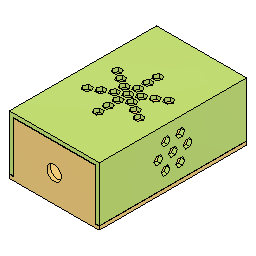
power-supply-case (Autodesk Fusion 360 design; units mm, degrees)
Autodesk Fusion 360 part; units mm, degrees
note: some values were not read from the file. Chosen so that the rebuilt part matches the saved one: which face or edge a step refers to. Set by a fixed rule: which sketch regions a step uses.
sketch "Sketch1" plane through (0, 0, 0) normal (0, 1, 0) x (1, 0, 0) in component "Bottom"
  line L0 (0, 0) -> (71, 0)
  line L1 (71, 0) -> (71, 116.4)
  line L2 (71, 116.4) -> (0, 116.4)
  line L3 (0, 116.4) -> (0, 0)
  dimension "d6" = 71
  dimension "d7" = 116.4
  dimension "d84" = 0
  dimension "d85" = 0
  dimension "d86" = 0
  dimension "d87" = 0
  constraint horizontal L0
  constraint vertical L1
  constraint horizontal L2
  constraint vertical L3
  constraint coincident L0.start L3.end
  measures "d6" distance of L0.start L0.end
  measures "d7" distance of L0.start L2.end
extrude "Extrude1" add sketch "Sketch1" along normal blind 42.8 makes body 1 in component "Bottom"
shell "Shell1" thickness 2.8 removed faces 1 at (23.6667, 42.8, -38.8) on bodies 1 in component "Bottom"
sketch "Sketch2" plane through (0, 42.8, 0) normal (0, 1, 0) x (-1, 0, 0) in component "Bottom"
  line L0 (-2.8, -113.6) -> (-68.2, -113.6)
  line L1 (-68.2, -113.6) -> (-68.2, -2.8)
  line L2 (-68.2, -2.8) -> (-2.8, -2.8)
  line L3 (-2.8, -2.8) -> (-2.8, -113.6)
  line L4 (0, -116.4) -> (0, 0)
  line L5 (0, 0) -> (-71, 0)
  line L6 (-71, 0) -> (-71, -116.4)
  line L7 (-71, -116.4) -> (0, -116.4)
  line L8 (0, -58.2) -> (-35.5, -58.2) construction
  line L9 (-67.9, 0) -> (-3.1, 0)
  line L10 (-3.1, 0) -> (-3.1, -116.4)
  line L11 (-3.1, -116.4) -> (-67.9, -116.4)
  line L12 (-67.9, -116.4) -> (-67.9, 0)
  line L13 (-67.9, 0) -> (-3.1, -116.4) construction
  line L14 (-3.1, 0) -> (-67.9, -116.4) construction
  point P0 (-35.5, -58.2)
  dimension "d11" = 35.5
  dimension "d12" = 116.4
  dimension "d13" = 64.8
  constraint horizontal L8
  constraint midpoint L4 L8.start
  constraint perpendicular L9 L10
  constraint parallel L9 L11
  constraint parallel L10 L12
  constraint horizontal L9
  constraint coincident L13 P0
  constraint coincident L14 P0
  constraint coincident P0 L8.end
  measures "d11" distance of L8.start P0
  measures "d12" distance of L9.end L10.end
  measures "d13" distance of L10.end L11.end
extrude "Extrude2" cut sketch "Sketch2" against normal blind 40 contours L0 L2 L3 L4 L5 L7 L10 | L0 L1 L2 L5 L6 L7 L12 bodies 1 in component "Bottom"
sketch "Sketch1 (2)" plane through (0, 42.8, 0) normal (0, 1, 0) x (-1, 0, 0) in component "Cover"
  line L0 (-3.1, -2.8) -> (-3.1, 0)
  line L1 (-3.1, 0) -> (-67.9, 0)
  line L2 (-67.9, 0) -> (-67.9, -2.8)
  line L3 (-67.9, -2.8) -> (-3.1, -2.8)
  line L4 (0, 0) -> (-71, 0)
  line L5 (-71, 0) -> (-71, -116)
  line L6 (-71, -116) -> (0, -116)
  line L7 (0, -116) -> (0, 0)
  dimension "d16" = 116
  dimension "d17" = 71
  dimension "d80" = 0
  dimension "d81" = 0
  dimension "d82" = 0
  dimension "d83" = 0
  constraint horizontal L4
  constraint vertical L5
  constraint horizontal L6
  constraint vertical L7
  constraint coincident L4.start L7.end
  measures "d16" distance of L4.start L6.end
  measures "d17" distance of L4.start L4.end
extrude "Extrude1'" add sketch "Sketch1 (2)" along normal blind 3 separate body makes body 2 in component "Cover"
sketch "Sketch2 (2)" plane through (0, 42.8, 0) normal (0, -1, 0) x (1, 0, 0) in component "Cover"
  line L0 (0, 0) -> (0, -116)
  line L1 (0, -116) -> (71, -116)
  line L2 (71, -116) -> (71, 0)
  line L3 (71, 0) -> (0, 0)
  line L4 (0, 0) -> (3, 0)
  line L5 (3, 0) -> (3, -116)
  line L6 (3, -116) -> (0, -116)
  line L7 (0, -116) -> (0, 0)
  line L8 (71, 0) -> (68, 0)
  line L9 (68, 0) -> (68, -116)
  line L10 (68, -116) -> (71, -116)
  line L11 (71, -116) -> (71, 0)
  dimension "d20" = 116
  dimension "d21" = 3
  dimension "d22" = 3
  dimension "d23" = 116
  constraint horizontal L4
  constraint vertical L5
  constraint horizontal L6
  constraint vertical L7
  constraint coincident L0.start L3.end
  constraint horizontal L8
  constraint vertical L9
  constraint horizontal L10
  constraint vertical L11
  constraint coincident L2.end L3.start
  measures "d20" distance of L0.start L0.end
  measures "d21" distance of L0.start L4.end
  measures "d22" distance of L2.end L8.end
  measures "d23" distance of L2.end L1.end
extrude "Extrude2'" add sketch "Sketch2 (2)" along normal blind 40 contours L0 L1 L3 L4 L5 L6 L7 | L1 L2 L3 L8 L9 L10 L11 bodies 2 in component "Cover"
sketch "Sketch2 (3)" plane through (68, 0, 0) normal (-1, 0, 0) x (0, 0, 1) in component "Cover"
  line L0 (0, 42.8) -> (-116, 42.8)
  line L1 (-116, 42.8) -> (-116, 2.8)
  line L2 (-116, 2.8) -> (0, 2.8)
  line L3 (0, 2.8) -> (0, 42.8)
  line L4 (-116, 42.8) -> (-113, 42.8) construction
  line L5 (-113, 42.8) -> (-110, 42.8)
  line L6 (-110, 42.8) -> (-110, 2.8)
  line L7 (-110, 2.8) -> (-113, 2.8)
  line L8 (-113, 2.8) -> (-113, 42.8)
  dimension "d26" = 3
  dimension "d27" = 3
  dimension "d28" = 40
  constraint coincident L0.end L1.start
  constraint perpendicular L1 L4
  constraint horizontal L5
  constraint vertical L6
  constraint horizontal L7
  constraint vertical L8
  measures "d26" distance of L0.end L4.end
  measures "d27" distance of L4.end L5.end
  measures "d28" distance of L4.end L7.end
extrude "Extrude3" add sketch "Sketch2 (3)" along normal blind 6 contours L0 L2 L5 L6 L7 L8 bodies 2 in component "Cover"
ref_plane "WorkPlane1" through (35.5, 24.3, -58) normal (0, 0, -1) x (-1, 0, 0) in component "Cover"
ref_plane "WorkPlane1" through (35.5, 22.8, -58) normal (-1, 0, 0) x (0, 0, -1) in component "Cover"
mirror "Mirror1" about plane through (35.5, 24.3, -58) normal (0, 0, -1) of "Extrude3" in component "Cover"
mirror "Mirror2" about plane through (35.5, 22.8, -58) normal (-1, 0, 0) of 6 faces at (62, 29.4667, -112) (66, 16.1333, -113) (66, 29.4667, -110) (66, 16.1333, -3) (62, 29.4667, -4) (66, 29.4667, -6) on bodies 2 in component "Cover"
chamfer "Chamfer1" distance 3 angle 45 2 edges at (68, 42.8, -58) (3, 42.8, -58) on bodies 2 in component "Cover"
chamfer "Chamfer2" distance 6 angle 45 4 edges at (68, 21.3, -6) (68, 21.3, -110) (3, 21.3, -110) (3, 21.3, -6) on bodies 2 in component "Cover"
chamfer "Chamfer1'" distance 3 angle 45 1 edges at (35.5, 2.8, -113.6) on bodies 1 in component "Bottom"
sketch "Sketch2 (1)" plane through (3.1, 0, 0) normal (-1, 0, 0) x (0, 0, 1) in component "Bottom"
  line L0 (-113.6, 5.8) -> (-113.6, 42.8)
  line L1 (-113.6, 42.8) -> (-116.4, 42.8)
  line L2 (-116.4, 2.8) -> (-110.6, 2.8)
  line L3 (-110.6, 2.8) -> (-113.6, 5.8)
  line L4 (-113.6, 5.8) -> (-113.6, 2.8)
  line L5 (-116.4, 42.8) -> (-116.4, 2.8)
  dimension "d36" = 3
  constraint vertical L4
  constraint coincident L0.start L3.end
  measures "d36" distance of L0.start L4.end
extrude "Extrude3'" cut sketch "Sketch2 (1)" against normal blind 7.5 contours L2 L3 L4 bodies 1 in component "Bottom"
sketch "Sketch3" plane through (67.9, 0, 0) normal (1, 0, 0) x (0, 0, -1) in component "Bottom"
  line L0 (110.6, 2.8) -> (116.4, 2.8)
  line L1 (116.4, 42.8) -> (113.6, 42.8)
  line L2 (113.6, 42.8) -> (113.6, 5.8)
  line L3 (113.6, 5.8) -> (110.6, 2.8)
  line L4 (113.6, 5.8) -> (113.6, 2.8)
  line L5 (116.4, 2.8) -> (116.4, 42.8)
  dimension "d39" = 3
  constraint vertical L4
  constraint coincident L2.end L3.start
  measures "d39" distance of L2.end L4.end
extrude "Extrude4" cut sketch "Sketch3" against normal blind 7.5 contours L0 L3 L4 bodies 1 in component "Bottom"
ref_plane "WorkPlane1" through (35.5, 22.8, -58.2) normal (0, 0, 1) x (1, 0, 0) in component "Bottom"
mirror "Mirror1'" about plane through (35.5, 22.8, -58.2) normal (0, 0, 1) of 3 faces at (43.8, 3.8, -111.6) (10.6, 3.8, -112.6) (60.4, 3.8, -112.6) on bodies 1 in component "Bottom"
sketch "Sketch4" plane through (0, 0, -116.4) normal (0, 0, -1) x (-1, 0, 0) in component "Bottom"
  line L0 (0, 2.8) -> (-3.1, 2.8)
  line L1 (-3.1, 2.8) -> (-3.1, 42.8)
  line L2 (-3.1, 42.8) -> (-67.9, 42.8)
  line L3 (-67.9, 42.8) -> (-67.9, 2.8)
  line L4 (-67.9, 2.8) -> (-71, 2.8)
  line L5 (-71, 2.8) -> (-71, 0)
  line L6 (-71, 0) -> (0, 0)
  line L7 (0, 0) -> (0, 2.8)
  line L8 (-18, 15.3) -> (-53, 15.3) construction
  line L9 (-53, 15.3) -> (-53, 30.3) construction
  line L10 (-53, 30.3) -> (-18, 30.3) construction
  line L11 (-18, 30.3) -> (-18, 15.3) construction
  line L12 (-18, 15.3) -> (-53, 30.3) construction
  line L13 (-53, 15.3) -> (-18, 30.3) construction
  line L14 (-30.4, 16.8) -> (-40.6, 16.8)
  line L15 (-45.6, 21.8) -> (-45.6, 23.8)
  line L16 (-40.6, 28.8) -> (-30.4, 28.8)
  line L17 (-25.4, 23.8) -> (-25.4, 21.8)
  line L18 (-25.4, 16.8) -> (-45.6, 28.8) construction
  line L19 (-45.6, 16.8) -> (-25.4, 28.8) construction
  arc A0 (-40.6, 28.8) -> (-45.6, 23.8) centre (-40.6, 23.8) ccw
  arc A1 (-25.4, 23.8) -> (-30.4, 28.8) centre (-30.4, 23.8) ccw
  arc A2 (-30.4, 16.8) -> (-25.4, 21.8) centre (-30.4, 21.8) ccw
  arc A3 (-45.6, 21.8) -> (-40.6, 16.8) centre (-40.6, 21.8) ccw
  line L20 (-67.9, 22.8) -> (-3.1, 22.8) construction
  point P0 (-35.5, 22.8)
  point P1 (-35.5, 22.8)
  dimension "d100" = 35
  dimension "d101" = 15
  dimension "d103" = 20.2
  dimension "d104" = 12
  dimension "d105" = 5
  constraint perpendicular L8 L9
  constraint parallel L8 L10
  constraint parallel L9 L11
  constraint horizontal L8
  constraint coincident L12 P1
  constraint coincident L13 P1
  constraint perpendicular L14 L15
  constraint parallel L14 L16
  constraint parallel L15 L17
  constraint horizontal L14
  constraint coincident L18 P1
  constraint coincident L19 P1
  constraint coincident P1 P0
  constraint coincident L18.end L15
  constraint coincident L18.end L16
  constraint tangent L15 A0
  constraint tangent L16 A0
  constraint coincident L19.end L16
  constraint coincident L19.end L17
  constraint tangent L16 A1
  constraint tangent L17 A1
  constraint equal A0 A1
  constraint coincident L18.start L14
  constraint coincident L18.start L17
  constraint tangent L14 A2
  constraint tangent L17 A2
  constraint equal A0 A2
  constraint coincident L19.start L14
  constraint coincident L19.start L15
  constraint tangent L14 A3
  constraint tangent L15 A3
  constraint equal A0 A3
  constraint midpoint L3 L20.start
  constraint midpoint L1 L20.end
  constraint midpoint P1 L20
  measures "d100" distance of L9.end L10.end
  measures "d101" distance of L8.end L9.end
  measures "d103" distance of L18.end L19.end
  measures "d104" distance of L19.start L18.end
  measures "d105" radius of A0
extrude "Extrude5" cut sketch "Sketch4" against normal up to surface (2.8 mm away) contours L14 L15 L16 L17 A0 A1 A2 A3 bodies 1 in component "Bottom"
sketch "Sketch3 (2)" plane through (0, 45.8, 0) normal (0, 1, 0) x (-1, 0, 0) in component "Cover"
  line L0 (0, -116) -> (0, 0)
  line L1 (0, 0) -> (-71, 0)
  line L2 (-71, 0) -> (-71, -116)
  line L3 (-71, -116) -> (0, -116)
  line L4 (-71, -58) -> (0, -58) construction
  line L5 (-35.5, -116) -> (-35.5, 0) construction
  line L6 (-38.9641, -58) -> (-37.2321, -61)
  line L7 (-37.2321, -61) -> (-33.7679, -61)
  line L8 (-33.7679, -61) -> (-32.0359, -58)
  line L9 (-32.0359, -58) -> (-33.7679, -55)
  line L10 (-33.7679, -55) -> (-37.2321, -55)
  line L11 (-37.2321, -55) -> (-38.9641, -58)
  line L12 (-38.0981, -59.5) -> (-40.6727, -60.9864) construction
  line L13 (-13.4164, -49.25) -> (-11.6843, -46.25)
  line L14 (-16.8805, -49.25) -> (-13.4164, -49.25)
  line L15 (-18.6125, -46.25) -> (-16.8805, -49.25)
  line L16 (-16.8805, -43.25) -> (-18.6125, -46.25)
  line L17 (-13.4164, -43.25) -> (-16.8805, -43.25)
  line L18 (-11.6843, -46.25) -> (-13.4164, -43.25)
  line L19 (-20.2002, -53.1667) -> (-18.4682, -50.1667)
  line L20 (-23.6643, -53.1667) -> (-20.2002, -53.1667)
  line L21 (-25.3964, -50.1667) -> (-23.6643, -53.1667)
  line L22 (-23.6643, -47.1667) -> (-25.3964, -50.1667)
  line L23 (-20.2002, -47.1667) -> (-23.6643, -47.1667)
  line L24 (-18.4682, -50.1667) -> (-20.2002, -47.1667)
  line L25 (-26.9841, -57.0833) -> (-25.252, -54.0833)
  line L26 (-30.4482, -57.0833) -> (-26.9841, -57.0833)
  line L27 (-32.1802, -54.0833) -> (-30.4482, -57.0833)
  line L28 (-30.4482, -51.0833) -> (-32.1802, -54.0833)
  line L29 (-26.9841, -51.0833) -> (-30.4482, -51.0833)
  line L30 (-25.252, -54.0833) -> (-26.9841, -51.0833)
  line L31 (-40.5518, -64.9167) -> (-38.8198, -61.9167)
  line L32 (-44.0159, -64.9167) -> (-40.5518, -64.9167)
  line L33 (-45.748, -61.9167) -> (-44.0159, -64.9167)
  line L34 (-44.0159, -58.9167) -> (-45.748, -61.9167)
  line L35 (-40.5518, -58.9167) -> (-44.0159, -58.9167)
  line L36 (-38.8198, -61.9167) -> (-40.5518, -58.9167)
  line L37 (-47.3357, -68.8333) -> (-45.6036, -65.8333)
  line L38 (-50.7998, -68.8333) -> (-47.3357, -68.8333)
  line L39 (-52.5318, -65.8333) -> (-50.7998, -68.8333)
  line L40 (-50.7998, -62.8333) -> (-52.5318, -65.8333)
  line L41 (-47.3357, -62.8333) -> (-50.7998, -62.8333)
  line L42 (-45.6036, -65.8333) -> (-47.3357, -62.8333)
  line L43 (-54.1195, -72.75) -> (-52.3875, -69.75)
  line L44 (-57.5836, -72.75) -> (-54.1195, -72.75)
  line L45 (-59.3157, -69.75) -> (-57.5836, -72.75)
  line L46 (-57.5836, -66.75) -> (-59.3157, -69.75)
  line L47 (-54.1195, -66.75) -> (-57.5836, -66.75)
  line L48 (-52.3875, -69.75) -> (-54.1195, -66.75)
  line L49 (-38.9641, -50.1667) -> (-37.2321, -53.1667)
  line L50 (-37.2321, -53.1667) -> (-33.7679, -53.1667)
  line L51 (-33.7679, -53.1667) -> (-32.0359, -50.1667)
  line L52 (-32.0359, -50.1667) -> (-33.7679, -47.1667)
  line L53 (-33.7679, -47.1667) -> (-37.2321, -47.1667)
  line L54 (-37.2321, -47.1667) -> (-38.9641, -50.1667)
  line L55 (-44.0159, -57.0833) -> (-40.5518, -57.0833)
  line L56 (-40.5518, -57.0833) -> (-38.8198, -54.0833)
  line L57 (-38.8198, -54.0833) -> (-40.5518, -51.0833)
  line L58 (-40.5518, -51.0833) -> (-44.0159, -51.0833)
  line L59 (-44.0159, -51.0833) -> (-45.748, -54.0833)
  line L60 (-45.748, -54.0833) -> (-44.0159, -57.0833)
  line L61 (-40.5518, -64.9167) -> (-38.8198, -61.9167)
  line L62 (-38.8198, -61.9167) -> (-40.5518, -58.9167)
  line L63 (-40.5518, -58.9167) -> (-44.0159, -58.9167)
  line L64 (-44.0159, -58.9167) -> (-45.748, -61.9167)
  line L65 (-45.748, -61.9167) -> (-44.0159, -64.9167)
  line L66 (-44.0159, -64.9167) -> (-40.5518, -64.9167)
  line L67 (-32.0359, -65.8333) -> (-33.7679, -62.8333)
  line L68 (-33.7679, -62.8333) -> (-37.2321, -62.8333)
  line L69 (-37.2321, -62.8333) -> (-38.9641, -65.8333)
  line L70 (-38.9641, -65.8333) -> (-37.2321, -68.8333)
  line L71 (-37.2321, -68.8333) -> (-33.7679, -68.8333)
  line L72 (-33.7679, -68.8333) -> (-32.0359, -65.8333)
  line L73 (-26.9841, -58.9167) -> (-30.4482, -58.9167)
  line L74 (-30.4482, -58.9167) -> (-32.1802, -61.9167)
  line L75 (-32.1802, -61.9167) -> (-30.4482, -64.9167)
  line L76 (-30.4482, -64.9167) -> (-26.9841, -64.9167)
  line L77 (-26.9841, -64.9167) -> (-25.252, -61.9167)
  line L78 (-25.252, -61.9167) -> (-26.9841, -58.9167)
  line L79 (-33.7679, -45.3333) -> (-32.0359, -42.3333)
  line L80 (-32.0359, -42.3333) -> (-33.7679, -39.3333)
  line L81 (-33.7679, -39.3333) -> (-37.2321, -39.3333)
  line L82 (-37.2321, -39.3333) -> (-38.9641, -42.3333)
  line L83 (-38.9641, -42.3333) -> (-37.2321, -45.3333)
  line L84 (-37.2321, -45.3333) -> (-33.7679, -45.3333)
  line L85 (-45.6036, -50.1667) -> (-47.3357, -47.1667)
  line L86 (-47.3357, -47.1667) -> (-50.7998, -47.1667)
  line L87 (-50.7998, -47.1667) -> (-52.5318, -50.1667)
  line L88 (-52.5318, -50.1667) -> (-50.7998, -53.1667)
  line L89 (-50.7998, -53.1667) -> (-47.3357, -53.1667)
  line L90 (-47.3357, -53.1667) -> (-45.6036, -50.1667)
  line L91 (-47.3357, -62.8333) -> (-50.7998, -62.8333)
  line L92 (-50.7998, -62.8333) -> (-52.5318, -65.8333)
  line L93 (-52.5318, -65.8333) -> (-50.7998, -68.8333)
  line L94 (-50.7998, -68.8333) -> (-47.3357, -68.8333)
  line L95 (-47.3357, -68.8333) -> (-45.6036, -65.8333)
  line L96 (-45.6036, -65.8333) -> (-47.3357, -62.8333)
  line L97 (-37.2321, -70.6667) -> (-38.9641, -73.6667)
  line L98 (-38.9641, -73.6667) -> (-37.2321, -76.6667)
  line L99 (-37.2321, -76.6667) -> (-33.7679, -76.6667)
  line L100 (-33.7679, -76.6667) -> (-32.0359, -73.6667)
  line L101 (-32.0359, -73.6667) -> (-33.7679, -70.6667)
  line L102 (-33.7679, -70.6667) -> (-37.2321, -70.6667)
  line L103 (-25.3964, -65.8333) -> (-23.6643, -68.8333)
  line L104 (-23.6643, -68.8333) -> (-20.2002, -68.8333)
  line L105 (-20.2002, -68.8333) -> (-18.4682, -65.8333)
  line L106 (-18.4682, -65.8333) -> (-20.2002, -62.8333)
  line L107 (-20.2002, -62.8333) -> (-23.6643, -62.8333)
  line L108 (-23.6643, -62.8333) -> (-25.3964, -65.8333)
  line L109 (-33.7679, -37.5) -> (-32.0359, -34.5)
  line L110 (-37.2321, -37.5) -> (-33.7679, -37.5)
  line L111 (-32.0359, -34.5) -> (-33.7679, -31.5)
  line L112 (-33.7679, -31.5) -> (-37.2321, -31.5)
  line L113 (-37.2321, -31.5) -> (-38.9641, -34.5)
  line L114 (-38.9641, -34.5) -> (-37.2321, -37.5)
  line L115 (-52.3875, -46.25) -> (-54.1195, -43.25)
  line L116 (-54.1195, -49.25) -> (-52.3875, -46.25)
  line L117 (-54.1195, -43.25) -> (-57.5836, -43.25)
  line L118 (-57.5836, -43.25) -> (-59.3157, -46.25)
  line L119 (-59.3157, -46.25) -> (-57.5836, -49.25)
  line L120 (-57.5836, -49.25) -> (-54.1195, -49.25)
  line L121 (-54.1195, -66.75) -> (-57.5836, -66.75)
  line L122 (-52.3875, -69.75) -> (-54.1195, -66.75)
  line L123 (-57.5836, -66.75) -> (-59.3157, -69.75)
  line L124 (-59.3157, -69.75) -> (-57.5836, -72.75)
  line L125 (-57.5836, -72.75) -> (-54.1195, -72.75)
  line L126 (-54.1195, -72.75) -> (-52.3875, -69.75)
  line L127 (-37.2321, -78.5) -> (-38.9641, -81.5)
  line L128 (-33.7679, -78.5) -> (-37.2321, -78.5)
  line L129 (-38.9641, -81.5) -> (-37.2321, -84.5)
  line L130 (-37.2321, -84.5) -> (-33.7679, -84.5)
  line L131 (-33.7679, -84.5) -> (-32.0359, -81.5)
  line L132 (-32.0359, -81.5) -> (-33.7679, -78.5)
  line L133 (-18.6125, -69.75) -> (-16.8805, -72.75)
  line L134 (-16.8805, -66.75) -> (-18.6125, -69.75)
  line L135 (-16.8805, -72.75) -> (-13.4164, -72.75)
  line L136 (-13.4164, -72.75) -> (-11.6843, -69.75)
  line L137 (-11.6843, -69.75) -> (-13.4164, -66.75)
  line L138 (-13.4164, -66.75) -> (-16.8805, -66.75)
  point P0 (-35.5, -58)
  dimension "d65" = 3
  dimension "d71" = 23.5
  dimension "d72" = 0
  dimension "d74" = 360
  dimension "d76" = 360
  dimension "d78" = 360
  constraint midpoint L2 L4.start
  constraint midpoint L0 L4.end
  constraint midpoint L3 L5.start
  constraint midpoint L1 L5.end
  constraint midpoint L5 P0
  constraint parallel L4 L7
  constraint midpoint L6 L12.start
  constraint perpendicular L6 L12
  measures "d65" distance of P0 L11
extrude "Extrude4'" cut sketch "Sketch3 (2)" against normal up to surface (3 mm away) contours L6 L7 L8 L9 L10 L11 | L13 L14 L15 L16 L17 L18 | L19 L20 L21 L22 L23 L24 | L25 L26 L27 L28 L29 L30 | L31 L32 L33 L34 L35 L36 L61 L62 L63 L64 L65 L66 | L37 L38 L39 L40 L41 L42 L91 L92 L93 L94 L95 L96 | L43 L44 L45 L46 L47 L48 L121 L122 L123 L124 L125 L126 | L49 L50 L51 L52 L53 L54 | L55 L56 L57 L58 L59 L60 | L67 L68 L69 L70 L71 L72 | L73 L74 L75 L76 L77 L78 | L79 L80 L81 L82 L83 L84 | L85 L86 L87 L88 L89 L90 | L97 L98 L99 L100 L101 L102 | L103 L104 L105 L106 L107 L108 | L109 L110 L111 L112 L113 L114 | L115 L116 L117 L118 L119 L120 | L127 L128 L129 L130 L131 L132 | L133 L134 L135 L136 L137 L138 bodies 2 in component "Cover"
sketch "Sketch4 (2)" plane through (71, 0, 0) normal (1, 0, 0) x (0, 0, -1) in component "Cover"
  line L0 (0, 2.8) -> (116, 2.8)
  line L1 (116, 2.8) -> (116, 45.8)
  line L2 (116, 45.8) -> (0, 45.8)
  line L3 (0, 45.8) -> (0, 2.8)
  line L4 (0, 45.8) -> (116, 2.8) construction
  line L5 (63.8133, 34.2769) -> (52.2664, 34.323) construction
  line L6 (52.2664, 34.323) -> (46.4531, 24.3461) construction
  line L7 (46.4531, 24.3461) -> (52.1867, 14.3231) construction
  line L8 (52.1867, 14.3231) -> (63.7336, 14.277) construction
  line L9 (63.7336, 14.277) -> (69.5469, 24.2539) construction
  line L10 (69.5469, 24.2539) -> (63.8133, 34.2769) construction
  line L11 (49.9172, 24.3461) -> (48.1851, 27.3461)
  line L12 (48.1851, 27.3461) -> (44.721, 27.3461)
  line L13 (44.721, 27.3461) -> (42.989, 24.3461)
  line L14 (42.989, 24.3461) -> (44.721, 21.3461)
  line L15 (44.721, 21.3461) -> (48.1851, 21.3461)
  line L16 (48.1851, 21.3461) -> (49.9172, 24.3461)
  line L17 (55.7305, 34.323) -> (53.9985, 37.323)
  line L18 (53.9985, 37.323) -> (50.5344, 37.323)
  line L19 (50.5344, 37.323) -> (48.8023, 34.323)
  line L20 (48.8023, 34.323) -> (50.5344, 31.323)
  line L21 (50.5344, 31.323) -> (53.9985, 31.323)
  line L22 (53.9985, 31.323) -> (55.7305, 34.323)
  line L23 (67.2775, 34.2769) -> (65.5454, 37.2769)
  line L24 (65.5454, 37.2769) -> (62.0813, 37.2769)
  line L25 (62.0813, 37.2769) -> (60.3492, 34.2769)
  line L26 (60.3492, 34.2769) -> (62.0813, 31.2769)
  line L27 (62.0813, 31.2769) -> (65.5454, 31.2769)
  line L28 (65.5454, 31.2769) -> (67.2775, 34.2769)
  line L29 (73.011, 24.2539) -> (71.279, 27.2539)
  line L30 (71.279, 27.2539) -> (67.8149, 27.2539)
  line L31 (67.8149, 27.2539) -> (66.0828, 24.2539)
  line L32 (66.0828, 24.2539) -> (67.8149, 21.2539)
  line L33 (67.8149, 21.2539) -> (71.279, 21.2539)
  line L34 (71.279, 21.2539) -> (73.011, 24.2539)
  line L35 (67.1977, 14.277) -> (65.4656, 17.277)
  line L36 (65.4656, 17.277) -> (62.0015, 17.277)
  line L37 (62.0015, 17.277) -> (60.2695, 14.277)
  line L38 (60.2695, 14.277) -> (62.0015, 11.277)
  line L39 (62.0015, 11.277) -> (65.4656, 11.277)
  line L40 (65.4656, 11.277) -> (67.1977, 14.277)
  line L41 (55.6508, 14.3231) -> (53.9187, 17.3231)
  line L42 (53.9187, 17.3231) -> (50.4546, 17.3231)
  line L43 (50.4546, 17.3231) -> (48.7225, 14.3231)
  line L44 (48.7225, 14.3231) -> (50.4546, 11.3231)
  line L45 (50.4546, 11.3231) -> (53.9187, 11.3231)
  line L46 (53.9187, 11.3231) -> (55.6508, 14.3231)
  line L47 (61.4641, 24.3) -> (59.7321, 27.3)
  line L48 (59.7321, 27.3) -> (56.2679, 27.3)
  line L49 (56.2679, 27.3) -> (54.5359, 24.3)
  line L50 (54.5359, 24.3) -> (56.2679, 21.3)
  line L51 (56.2679, 21.3) -> (59.7321, 21.3)
  line L52 (59.7321, 21.3) -> (61.4641, 24.3)
  line L53 (0, 24.3) -> (116, 24.3) construction
  point P0 (58, 24.3)
  point P1 (46.4531, 24.3461)
  point P2 (52.2664, 34.323)
  point P3 (63.8133, 34.2769)
  point P4 (69.5469, 24.2539)
  point P5 (63.7336, 14.277)
  point P6 (52.1867, 14.3231)
  point P7 (58, 24.3)
  dimension "d53" = 10
  dimension "d54" = 3
  dimension "d55" = 3
  dimension "d56" = 3
  dimension "d57" = 3
  dimension "d58" = 3
  dimension "d59" = 3
  dimension "d60" = 3
  constraint coincident L2.end L3.start
  constraint coincident L0.end L1.start
  constraint midpoint L4 P7
  constraint coincident P1 L6.end
  constraint coincident P2 L5.end
  constraint coincident P3 L5.start
  constraint coincident P4 L9.end
  constraint coincident P5 L8.end
  constraint coincident P6 L7.end
  constraint coincident P7 P0
  constraint midpoint L3 L53.start
  constraint midpoint L1 L53.end
  constraint parallel L21 L53
  constraint parallel L27 L53
  constraint parallel L15 L53
  constraint parallel L51 L53
  constraint parallel L33 L53
  constraint parallel L45 L53
  constraint parallel L39 L53
  measures "d53" distance of P7 L10
  measures "d54" distance of P1 L16
  measures "d55" distance of P2 L22
  measures "d56" distance of P3 L28
  measures "d57" distance of P4 L34
  measures "d58" distance of P5 L40
  measures "d59" distance of P6 L46
  measures "d60" distance of P7 L52
extrude "Extrude5'" cut sketch "Sketch4 (2)" against normal up to surface (3 mm away) contours L11 L12 L13 L14 L15 L16 | L17 L18 L19 L20 L21 L22 | L23 L24 L25 L26 L27 L28 | L29 L30 L31 L32 L33 L34 | L35 L36 L37 L38 L39 L40 | L41 L42 L43 L44 L45 L46 | L47 L48 L49 L50 L51 L52 bodies 2 in component "Cover"
sketch "Sketch5" plane through (0, 0, 0) normal (-1, 0, 0) x (0, 0, 1) in component "Cover"
  line L0 (-116, 2.8) -> (0, 2.8)
  line L1 (0, 2.8) -> (0, 45.8)
  line L2 (0, 45.8) -> (-116, 45.8)
  line L3 (-116, 45.8) -> (-116, 2.8)
  line L4 (-65.5454, 37.2769) -> (-62.0813, 37.2769)
  line L5 (-62.0813, 37.2769) -> (-60.3492, 34.2769)
  line L6 (-60.3492, 34.2769) -> (-62.0813, 31.2769)
  line L7 (-62.0813, 31.2769) -> (-65.5454, 31.2769)
  line L8 (-65.5454, 31.2769) -> (-67.2775, 34.2769)
  line L9 (-67.2775, 34.2769) -> (-65.5454, 37.2769)
  line L10 (-55.7305, 34.323) -> (-53.9985, 37.323)
  line L11 (-53.9985, 37.323) -> (-50.5344, 37.323)
  line L12 (-50.5344, 37.323) -> (-48.8023, 34.323)
  line L13 (-48.8023, 34.323) -> (-50.5344, 31.323)
  line L14 (-50.5344, 31.323) -> (-53.9985, 31.323)
  line L15 (-53.9985, 31.323) -> (-55.7305, 34.323)
  line L16 (-71.279, 27.2539) -> (-67.8149, 27.2539)
  line L17 (-73.011, 24.2539) -> (-71.279, 27.2539)
  line L18 (-71.279, 21.2539) -> (-73.011, 24.2539)
  line L19 (-67.8149, 21.2539) -> (-71.279, 21.2539)
  line L20 (-66.0828, 24.2539) -> (-67.8149, 21.2539)
  line L21 (-67.8149, 27.2539) -> (-66.0828, 24.2539)
  line L22 (-61.4641, 24.3) -> (-59.7321, 27.3)
  line L23 (-59.7321, 27.3) -> (-56.2679, 27.3)
  line L24 (-56.2679, 27.3) -> (-54.5359, 24.3)
  line L25 (-54.5359, 24.3) -> (-56.2679, 21.3)
  line L26 (-56.2679, 21.3) -> (-59.7321, 21.3)
  line L27 (-59.7321, 21.3) -> (-61.4641, 24.3)
  line L28 (-49.9172, 24.3461) -> (-48.1851, 27.3461)
  line L29 (-48.1851, 27.3461) -> (-44.721, 27.3461)
  line L30 (-44.721, 27.3461) -> (-42.989, 24.3461)
  line L31 (-42.989, 24.3461) -> (-44.721, 21.3461)
  line L32 (-44.721, 21.3461) -> (-48.1851, 21.3461)
  line L33 (-48.1851, 21.3461) -> (-49.9172, 24.3461)
  line L34 (-50.4546, 17.3231) -> (-48.7225, 14.3231)
  line L35 (-53.9187, 17.3231) -> (-50.4546, 17.3231)
  line L36 (-55.6508, 14.3231) -> (-53.9187, 17.3231)
  line L37 (-53.9187, 11.3231) -> (-55.6508, 14.3231)
  line L38 (-50.4546, 11.3231) -> (-53.9187, 11.3231)
  line L39 (-48.7225, 14.3231) -> (-50.4546, 11.3231)
  line L40 (-62.0015, 17.277) -> (-60.2695, 14.277)
  line L41 (-65.4656, 17.277) -> (-62.0015, 17.277)
  line L42 (-67.1977, 14.277) -> (-65.4656, 17.277)
  line L43 (-65.4656, 11.277) -> (-67.1977, 14.277)
  line L44 (-62.0015, 11.277) -> (-65.4656, 11.277)
  line L45 (-60.2695, 14.277) -> (-62.0015, 11.277)
extrude "Extrude6" cut sketch "Sketch5" against normal up to surface (3 mm away) contours L4 L5 L6 L7 L8 L9 | L10 L11 L12 L13 L14 L15 | L16 L17 L18 L19 L20 L21 | L22 L23 L24 L25 L26 L27 | L28 L29 L30 L31 L32 L33 | L34 L35 L36 L37 L38 L39 | L40 L41 L42 L43 L44 L45 bodies 2 in component "Cover"
sketch "Sketch5 (2)" plane through (0, 0, 0) normal (0, 0, 1) x (1, 0, 0) in component "Bottom"
  line L0 (0, 0) -> (71, 0)
  line L1 (71, 0) -> (71, 2.8)
  line L2 (71, 2.8) -> (67.9, 2.8)
  line L3 (67.9, 2.8) -> (67.9, 42.8)
  line L4 (67.9, 42.8) -> (3.1, 42.8)
  line L5 (3.1, 42.8) -> (3.1, 2.8)
  line L6 (3.1, 2.8) -> (0, 2.8)
  line L7 (0, 2.8) -> (0, 0)
  line L8 (35.5, 42.8) -> (35.5, 0) construction
  circle A0 centre (35.5, 21.4) radius 5.7
  dimension "d109" = 11.4
  constraint midpoint L4 L8.start
  constraint midpoint L0 L8.end
  constraint midpoint L8 A0.centre
  measures "d109" diameter of A0
extrude "Extrude6'" cut sketch "Sketch5 (2)" against normal up to surface (2.8 mm away) contours A0 bodies 1 in component "Bottom"
component "Bottom" placed x (1, 0, 0) y (0, 1, 0) z (0, 0, 1) at (0, 0, 0)
component "Cover" placed x (1, 0, 0) y (0, 1, 0) z (0, 0, 1) at (0, 0.2, -0.2)
equation "devLength = 110 mm"
equation "devWidth = 65 mm"
equation "devHeight = 40 mm"
equation "wallThickness = 3 mm"
equation "tolerance = 0.2 mm"
equation "d6 = devWidth + wallThickness * 2"
equation "d7 = devLength + ( wallThickness * 2 ) + ( tolerance * 2 )"
equation "d8 = devHeight + wallThickness - tolerance"
equation "d10 = wallThickness - tolerance"
equation "d11 = devWidth / 2 + wallThickness"
equation "d12 = devLength + ( wallThickness * 2 ) + ( tolerance * 2 )"
equation "d13 = devWidth - tolerance"
equation "d14 = -devHeight"
equation "d16 = devLength + wallThickness * 2"
equation "d17 = devWidth + wallThickness * 2"
equation "d18 = wallThickness"
equation "d20 = devLength + wallThickness * 2"
equation "d21 = wallThickness"
equation "d22 = wallThickness"
equation "d23 = devLength + wallThickness * 2"
equation "d24 = devHeight"
equation "d26 = wallThickness"
equation "d27 = wallThickness"
equation "d28 = devHeight"
equation "d29 = wallThickness * 2"
equation "d33 = wallThickness"
equation "d34 = wallThickness * 2"
equation "d35 = wallThickness"
equation "d36 = wallThickness"
equation "d37 = -wallThickness * 2.5"
equation "d39 = wallThickness"
equation "d40 = -wallThickness * 2.5"
equation "d53 = devHeight / 4"
equation "d54 = wallThickness"
equation "d55 = wallThickness"
equation "d56 = wallThickness"
equation "d57 = wallThickness"
equation "d58 = wallThickness"
equation "d59 = wallThickness"
equation "d60 = wallThickness"
equation "d65 = wallThickness"
equation "d71 = devWidth / 2 - wallThickness * 3"
equation "d90 = -tolerance"
equation "dcConnDiam = 11.4 mm"
equation "d109 = dcConnDiam"
